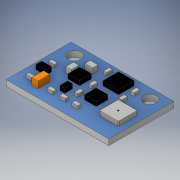
# Autodesk Inventor part: GY81
Saved by Autodesk Inventor 2016 (Build 200138000, 138)
## iProperties
Created: 2015-11-27
Part Number: GY81
Material: Generic
Document SubType Name: Modeling
Designer: Spooner
Density: 1 g/cm^3
Appearance: Default
Author: Spooner
Autodesk Inventor part; units mm, degrees
ref_plane "YZ Plane" through (0, 0, 0) normal (1, 0, 0) x (0, 1, 0)
ref_plane "XZ Plane" through (0, 0, 0) normal (0, 1, 0) x (-1, 0, 0)
ref_plane "XY Plane" through (0, 0, 0) normal (0, 0, 1) x (1, 0, 0)
sketch "Sketch1" plane through (0, 0, 0) normal (0, 1, 0) x (-1, 0, 0)
  line L0 (0, 0) -> (-26.67, 0)
  line L1 (-26.67, 0) -> (-26.67, -16.891)
  line L2 (-26.67, -16.891) -> (0, -16.891)
  line L3 (0, -16.891) -> (0, 0)
  circle A0 centre (-3.5369, -14.2431) radius 1.632
  circle A1 centre (-23.133, -14.2431) radius 1.632
  dimension "d0" = 16.891
  dimension "d1" = 26.67
  dimension "d2" = 3.2639
  dimension "d3" = 1.016
  dimension "d4" = 1.905
  dimension "d5" = 1.905
  constraints: 8 end point, 2 centre point, 2 parallel, 1 equal radius, 1 horizontal, 1 horizontal alignment, 1 perpendicular
  measures "d0" distance of L2.end L0.start
  measures "d1" distance of L1.end L2.end
  measures "d2" diameter of A0
  measures "d3" distance edge to line of A0 L2
  measures "d4" distance edge to line of A0 L3
  measures "d5" distance edge to line of A1 L1
extrude "Board" add sketch "Sketch1" along normal blind 1.524
sketch "Sketch2" plane through (0, 1.524, 0) normal (0, 1, 0) x (1, 0, 0)
  line L0 (20.1803, 4.0513) -> (25.0698, 4.0513)
  line L1 (25.0698, 4.0513) -> (25.0698, 8.9408)
  line L2 (25.0698, 8.9408) -> (20.1803, 8.9408)
  line L3 (20.1803, 8.9408) -> (20.1803, 4.0513)
  line L4 (26.67, 0) -> (26.67, 16.891) projected
  line L5 (26.67, 16.891) -> (0, 16.891) projected
  point P0 (0, 0)
  dimension "d8" = 4.8895
  dimension "d9" = 1.6002
  dimension "d10" = 7.9502
  constraints: 8 end point, 2 parallel, 2 perpendicular, 1 horizontal
  measures "d8" distance of L0.start L0.end
  measures "d9" distance between parallel lines of L4 L1
  measures "d10" distance between parallel lines of L2 L5
extrude "BMP085 Barometer" add sketch "Sketch2" along normal blind 1.1176
fillet "BMP085 Barometer Fillets" radius 0.254 4 edges at (25.0698, 2.0828, -4.0513) (20.1803, 2.0828, -4.0513) (20.1803, 2.0828, -8.9408) (25.0698, 2.0828, -8.9408)
sketch "Sketch3" plane through (0, 2.6416, 0) normal (0, 1, 0) x (1, 0, 0)
  circle A0 centre (22.6251, 6.4961) radius 0.1905
  line L0 (24.8158, 8.9408) -> (20.4343, 8.9408) projected
  line L1 (20.1803, 8.6868) -> (20.1803, 4.3053) projected
  point P0 (0, 0)
  point P1 (22.6251, 8.9408)
  point P2 (20.1803, 6.4961)
  dimension "d14" = 0.381
  constraints: 2 midpoint, 1 centre point, 1 horizontal alignment, 1 vertical alignment
  measures "d14" diameter of A0
extrude "BMP085 Barometer Hole" cut sketch "Sketch3" against normal blind 0.0254
sketch "Sketch4" plane through (0, 1.524, 0) normal (0, 1, 0) x (1, 0, 0)
  line L0 (13.97, 15.24) -> (18.034, 15.24)
  line L1 (18.034, 15.24) -> (18.034, 11.176)
  line L2 (18.034, 11.176) -> (13.97, 11.176)
  line L3 (13.97, 11.176) -> (13.97, 15.24)
  line L4 (14.7193, 8.6868) -> (17.7673, 8.6868)
  line L5 (17.7673, 8.6868) -> (17.7673, 5.6388)
  line L6 (17.7673, 5.6388) -> (14.7193, 5.6388)
  line L7 (14.7193, 5.6388) -> (14.7193, 8.6868)
  line L8 (7.874, 11.2141) -> (10.922, 11.2141)
  line L9 (10.922, 11.2141) -> (10.922, 8.1661)
  line L10 (10.922, 8.1661) -> (7.874, 8.1661)
  line L11 (7.874, 8.1661) -> (7.874, 11.2141)
  line L12 (9.4361, 6.5532) -> (10.7061, 6.5532)
  line L13 (10.7061, 6.5532) -> (10.7061, 4.5212)
  line L14 (10.7061, 4.5212) -> (9.4361, 4.5212)
  line L15 (9.4361, 4.5212) -> (9.4361, 6.5532)
  line L16 (1.6129, 7.6581) -> (4.1529, 7.6581)
  line L17 (4.1529, 7.6581) -> (4.1529, 6.1341)
  line L18 (4.1529, 6.1341) -> (1.6129, 6.1341)
  line L19 (1.6129, 6.1341) -> (1.6129, 7.6581)
  line L20 (26.67, 16.891) -> (0, 16.891) projected
  line L21 (26.67, 0) -> (26.67, 16.891) projected
  line L22 (20.1803, 4.3053) -> (20.1803, 8.6868) projected
  line L23 (0, 16.891) -> (0, 0) projected
  dimension "d17" = 4.064
  dimension "d18" = 3.048
  dimension "d19" = 1.27
  dimension "d20" = 2.032
  dimension "d21" = 1.524
  dimension "d22" = 2.54
  dimension "d23" = 1.651
  dimension "d24" = 8.636
  dimension "d25" = 2.413
  dimension "d26" = 2.4892
  dimension "d27" = 3.048
  dimension "d28" = 5.6769
  dimension "d29" = 4.0132
  dimension "d30" = 1.6129
  dimension "d31" = 1.6129
  dimension "d32" = 9.2329
  constraints: 40 end point, 10 parallel, 5 horizontal, 5 perpendicular, 4 equal length
  measures "d17" distance of L0.start L0.end
  measures "d18" distance of L4.start L4.end
  measures "d19" distance of L12.start L12.end
  measures "d20" distance of L14.end L12.start
  measures "d21" distance of L18.end L16.start
  measures "d22" distance of L16.start L16.end
  measures "d23" distance between parallel lines of L20 L0
  measures "d24" distance between parallel lines of L21 L1
  measures "d25" distance between parallel lines of L22 L5
  measures "d26" distance between parallel lines of L2 L4
  measures "d27" distance between parallel lines of L3 L9
  measures "d28" distance between parallel lines of L20 L8
  measures "d29" distance between parallel lines of L7 L13
  measures "d30" distance between parallel lines of L10 L12
  measures "d31" distance between parallel lines of L23 L19
  measures "d32" distance between parallel lines of L16 L20
extrude "Extrusion4" add sketch "Sketch4" along normal blind 1.1684
sketch "Sketch5" plane through (0, 1.524, 0) normal (0, 1, 0) x (1, 0, 0)
  line L0 (4.5925, 5.1224) -> (6.2054, 5.1224)
  line L1 (6.2054, 5.1224) -> (6.2054, 2.0744)
  line L2 (6.2054, 2.0744) -> (4.5925, 2.0744)
  line L3 (4.5925, 2.0744) -> (4.5925, 5.1224)
  point P0 (0, 0)
  dimension "d35" = 1.6129
  dimension "d36" = 3.048
  constraints: 8 end point, 2 parallel, 1 horizontal, 1 perpendicular
  measures "d35" distance of L1.end L2.end
  measures "d36" distance of L2.end L0.start
extrude "Extrusion5" add sketch "Sketch5" along normal blind 1.7399
sketch "Sketch6" plane through (0, 1.524, 0) normal (0, 1, 0) x (1, 0, 0)
  line L0 (8.0137, 13.843) -> (9.9949, 13.843)
  line L1 (9.9949, 13.843) -> (9.9949, 12.446)
  line L2 (9.9949, 12.446) -> (8.0137, 12.446)
  line L3 (8.0137, 12.446) -> (8.0137, 13.843)
  line L4 (0, 16.891) -> (0, 0) projected
  line L5 (6.2357, 11.2649) -> (7.6327, 11.2649)
  line L6 (7.6327, 11.2649) -> (7.6327, 9.2837)
  line L7 (7.6327, 9.2837) -> (6.2357, 9.2837)
  line L8 (6.2357, 9.2837) -> (6.2357, 11.2649)
  line L9 (26.67, 16.891) -> (0, 16.891) projected
  dimension "d39" = 1.9812
  dimension "d41" = 8.0137
  dimension "d42" = 1.397
  dimension "d43" = 6.2357
  dimension "d44" = 3.048
  dimension "d45" = 5.6261
  constraints: 16 end point, 4 parallel, 4 perpendicular, 2 horizontal
  measures "d39" distance of L0.start L0.end
  measures "d41" distance between parallel lines of L4 L3
  measures "d42" distance of L5.start L5.end
  measures "d43" distance between parallel lines of L4 L8
  measures "d44" distance between parallel lines of L0 L9
  measures "d45" distance between parallel lines of L5 L9
extrude "Extrusion6" add sketch "Sketch6" along normal blind 1.397
sketch "Sketch7" plane through (0, 1.524, 0) normal (0, 1, 0) x (1, 0, 0)
  line L0 (19.4691, 14.3256) -> (20.3708, 14.3256)
  line L1 (20.3708, 14.3256) -> (20.3708, 12.8397)
  line L2 (20.3708, 12.8397) -> (19.4691, 12.8397)
  line L3 (19.4691, 12.8397) -> (19.4691, 14.3256)
  line L4 (19.4691, 11.176) -> (20.3708, 11.176)
  line L5 (20.3708, 11.176) -> (20.3708, 9.6901)
  line L6 (20.3708, 9.6901) -> (19.4691, 9.6901)
  line L7 (19.4691, 9.6901) -> (19.4691, 11.176)
  line L8 (11.43, 15.3162) -> (12.2809, 15.3162)
  line L9 (12.2809, 15.3162) -> (12.2809, 13.8303)
  line L10 (12.2809, 13.8303) -> (11.43, 13.8303)
  line L11 (11.43, 13.8303) -> (11.43, 15.3162)
  line L12 (12.4206, 10.4902) -> (13.3223, 10.4902)
  line L13 (13.3223, 10.4902) -> (13.3223, 9.0043)
  line L14 (13.3223, 9.0043) -> (12.4206, 9.0043)
  line L15 (12.4206, 9.0043) -> (12.4206, 10.4902)
  line L16 (12.4206, 6.8072) -> (13.3223, 6.8072)
  line L17 (13.3223, 6.8072) -> (13.3223, 5.3213)
  line L18 (13.3223, 5.3213) -> (12.4206, 5.3213)
  line L19 (12.4206, 5.3213) -> (12.4206, 6.8072)
  line L20 (8.0215, 3.5052) -> (9.5074, 3.5052)
  line L21 (9.5074, 3.5052) -> (9.5074, 2.6035)
  line L22 (9.5074, 2.6035) -> (8.0215, 2.6035)
  line L23 (8.0215, 2.6035) -> (8.0215, 3.5052)
  line L24 (11.26, 3.5052) -> (12.7459, 3.5052)
  line L25 (12.7459, 3.5052) -> (12.7459, 2.6035)
  line L26 (12.7459, 2.6035) -> (11.26, 2.6035)
  line L27 (11.26, 2.6035) -> (11.26, 3.5052)
  line L28 (14.4985, 3.5052) -> (15.9844, 3.5052)
  line L29 (15.9844, 3.5052) -> (15.9844, 2.6035)
  line L30 (15.9844, 2.6035) -> (14.4985, 2.6035)
  line L31 (14.4985, 2.6035) -> (14.4985, 3.5052)
  line L32 (26.67, 16.891) -> (0, 16.891) projected
  line L33 (9.4361, 4.5212) -> (10.7061, 4.5212) projected
  line L34 (2.159, 9.6901) -> (3.6449, 9.6901)
  line L35 (3.6449, 9.6901) -> (3.6449, 8.8392)
  line L36 (3.6449, 8.8392) -> (2.159, 8.8392)
  line L37 (2.159, 8.8392) -> (2.159, 9.6901)
  line L38 (2.159, 3.81) -> (3.6449, 3.81)
  line L39 (3.6449, 3.81) -> (3.6449, 2.9591)
  line L40 (3.6449, 2.9591) -> (2.159, 2.9591)
  line L41 (2.159, 2.9591) -> (2.159, 3.81)
  line L42 (0, 16.891) -> (0, 0) projected
  line L43 (1.6129, 6.1341) -> (4.1529, 6.1341) projected
  line L44 (6.2054, 2.0744) -> (6.2054, 5.1224) projected
  line L45 (14.7193, 8.6868) -> (14.7193, 5.6388) projected
  line L46 (13.97, 15.24) -> (13.97, 11.176) projected
  line L47 (18.034, 11.176) -> (18.034, 15.24) projected
  point P0 (19.92, 12.8397)
  point P1 (19.92, 11.176)
  point P2 (12.8714, 9.0043)
  point P3 (12.8714, 6.8072)
  point P4 (2.159, 9.2647)
  point P5 (2.159, 3.3846)
  dimension "d48" = 0.8509
  dimension "d49" = 1.4859
  dimension "d50" = 1.5748
  dimension "d51" = 2.5654
  dimension "d52" = 1.6637
  dimension "d53" = 3.3401
  dimension "d54" = 2.1971
  dimension "d56" = 1.016
  dimension "d57" = 2.159
  dimension "d58" = 7.2009
  dimension "d59" = 2.3241
  dimension "d60" = 1.8161
  dimension "d61" = 1.7526
  dimension "d62" = 1.7526
  dimension "d63" = 0.9017
  dimension "d64" = 1.397
  dimension "d65" = 1.6891
  dimension "d66" = 1.4351
  constraints: 80 end point, 20 parallel, 14 equal length, 10 horizontal, 10 perpendicular, 7 point on line, 6 midpoint, 3 vertical alignment, 2 horizontal alignment
  measures "d48" distance of L8.start L8.end
  measures "d49" distance of L10.end L8.start
  measures "d50" distance between parallel lines of L32 L8
  measures "d51" distance between parallel lines of L0 L32
  measures "d52" distance of point (19.92, 12.84) point (19.92, 11.176)
  measures "d53" distance between parallel lines of L12 L10
  measures "d54" distance of point (12.871, 9.004) point (12.871, 6.807)
  measures "d56" distance between parallel lines of L33 L20
  measures "d57" distance from line of L42 point (2.159, 9.265)
  measures "d58" distance between parallel lines of L32 L34
  measures "d59" distance between parallel lines of L38 L43
  measures "d60" distance from line of L20.start L44
  measures "d61" distance between parallel lines of L27 L21
  measures "d62" distance between parallel lines of L31 L25
  measures "d63" distance of L29.end L28.end
  measures "d64" distance between parallel lines of L45 L17
  measures "d65" distance between parallel lines of L46 L9
  measures "d66" distance between parallel lines of L47 L3
extrude "Extrusion7" add sketch "Sketch7" along normal blind 0.762
equation "\"d5\" = d4"
equation "\"d62\" = d61"
body "Solid1"
